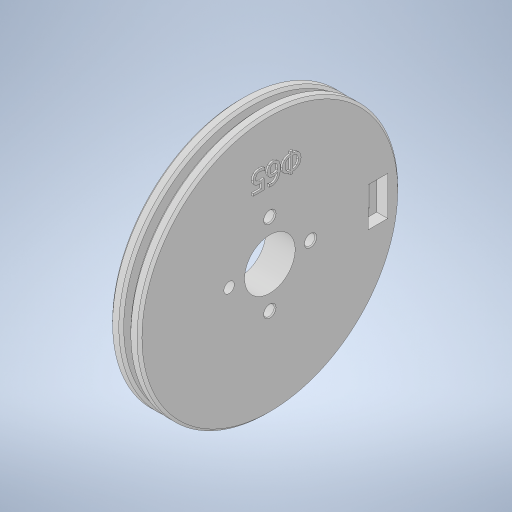
# Autodesk Inventor part: pully_elbow
Saved by Autodesk Inventor 2024 (Build 280153000, 153)
## iProperties
Created: 2025-06-10
Part Number: pully_elbow
Material: 一般
Document SubType Name: Modeling
Designer: HosodaLab2
Density: 1 g/cm^3
Appearance: 既定
Author: HosodaLab2
Autodesk Inventor part; units mm, degrees
ref_plane "YZ Plane" through (0, 0, 0) normal (1, 0, 0) x (0, 1, 0)
ref_plane "XZ Plane" through (0, 0, 0) normal (0, 1, 0) x (-1, 0, 0)
ref_plane "XY Plane" through (0, 0, 0) normal (0, 0, 1) x (1, 0, 0)
sketch "スケッチ1" plane through (0, 0, 0) normal (0, 1, 0) x (-1, 0, 0)
  circle A0 centre (0, 0) radius 32.5
  dimension "d0" = 65
  constraints: 1 centre point, 1 coincident
  measures "d0" diameter of A0
extrude "押し出し1" add sketch "スケッチ1" along normal blind 2.2
sketch "スケッチ2" plane through (0, 2.2, 0) normal (0, 1, 0) x (1, 0, 0)
  circle A0 centre (0, 0) radius 40
  line L0 (-3.103, -20.7113) -> (4.1548, -20.7113) construction
  line L1 (4.1548, -20.7113) -> (4.1548, -23.6986) construction
  line L2 (4.1548, -23.6986) -> (-3.103, -23.6986) construction
  line L3 (-3.103, -23.6986) -> (-3.103, -20.7113) construction
  dimension "d3" = 80
  constraints: 1 centre point, 1 coincident, 2 other
  measures "d3" diameter of A0
extrude "押し出し2" add sketch "スケッチ2" along normal blind 3.4
chamfer "面取り1" distance 0.75 angle 45 1 edges at (-40, 2.2, 0)
chamfer "面取り2" distance 0.75 angle 45 1 edges at (-40, 5.6, 0)
sketch "スケッチ3" plane through (0, 0, 0) normal (0, -1, 0) x (1, 0, 0)
  circle A0 centre (0, 0) radius 40
  dimension "d12" = 80
  constraints: 1 centre point, 1 coincident
  measures "d12" diameter of A0
extrude "押し出し3" add sketch "スケッチ3" along normal blind 3.4
chamfer "面取り3" distance 0.75 angle 45 1 edges at (-40, 0, 0)
chamfer "面取り4" distance 0.75 angle 45 1 edges at (-40, -3.4, 0)
sketch "スケッチ5" plane through (0, -3.4, 0) normal (0, -1, 0) x (1, 0, 0)
  circle A0 centre (0, 0) radius 12.5
  point P0 (0, -12.5)
  point P1 (0, 12.5)
  point P2 (-12.5, 0)
  point P3 (12.5, 0)
  dimension "d30" = 25
  constraints: 4 point on circle, 1 centre point, 1 coincident
  measures "d30" diameter of A0
hole "穴1" at (0, -3.4, -12.5) at (0, -3.4, 12.5) at (-12.5, -3.4, 0) at (12.5, -3.4, 0) direction (0, 1, 0) diameter 3.2 end through all
fillet "フィレット1" radius 0.3 6 edges at (0, -3.4, -10.9) (-12.5, -3.4, 1.6) (0, -3.4, 14.1) (0, 5.6, -10.9) (-12.5, 5.6, 1.6) (0, 5.6, 14.1)
sketch "スケッチ6" plane through (0, 5.6, 0) normal (0, 1, 0) x (1, 0, 0)
  circle A0 centre (0, 0) radius 3.15
  line L0 (0, 3.15) -> (39.8758, 3.15)
  circle A1 centre (0, 0) radius 40 projected
  line L1 (0, -3.15) -> (39.8758, -3.15)
  dimension "d39" = 6.3
  constraints: 4 end point, 4 point on circle, 1 centre point, 1 coincident, 1 horizontal, 1 parallel, 1 tangent
  measures "d39" diameter of A0
extrude "押し出し5" [suppressed]
chamfer "面取り7" [suppressed]
chamfer "面取り8" [suppressed]
chamfer "面取り9" [suppressed]
sketch "スケッチ7" plane through (0, 5.6, 0) normal (0, 1, 0) x (1, 0, 0)
  line L0 (-9.3358, -20.9354) -> (21.308, -20.9354) construction
  line L1 (21.308, -20.9354) -> (21.308, -27.5341) construction
  line L2 (21.308, -27.5341) -> (-9.3358, -27.5341) construction
  line L3 (-9.3358, -27.5341) -> (-9.3358, -20.9354) construction
  spline S0 degree 2 poles (-5.7914, -21.6472) (-5.2131, -21.6571) (-4.2541, -22.0427) (-3.9377, -22.364) knots 0 0 0 1 2 2 2
  spline S1 degree 2 poles (-3.9377, -22.364) (-3.646, -22.6655) (-3.3247, -23.5108) (-3.3247, -24.0546) knots 0 0 0 1 2 2 2
  spline S2 degree 2 poles (-3.3247, -24.0546) (-3.3247, -24.6231) (-3.6708, -25.498) (-3.9772, -25.7946) knots 0 0 0 1 2 2 2
  spline S3 degree 2 poles (-3.9772, -25.7946) (-4.3084, -26.1209) (-5.2773, -26.4818) (-5.7914, -26.4916) knots 0 0 0 1 2 2 2
  line L4 (-5.7914, -26.4916) -> (-5.7914, -27.1985)
  line L5 (-5.7914, -27.1985) -> (-6.6021, -27.1985)
  line L6 (-6.6021, -27.1985) -> (-6.6021, -26.4916)
  spline S4 degree 2 poles (-6.6021, -26.4916) (-7.1162, -26.4768) (-8.0802, -26.1407) (-8.4213, -25.8045) knots 0 0 0 1 2 2 2
  spline S5 degree 2 poles (-8.4213, -25.8045) (-8.7277, -25.503) (-9.0688, -24.6181) (-9.0688, -24.0546) knots 0 0 0 1 2 2 2
  spline S6 degree 2 poles (-9.0688, -24.0546) (-9.0688, -23.5207) (-8.7426, -22.6754) (-8.446, -22.369) knots 0 0 0 1 2 2 2
  spline S7 degree 2 poles (-8.446, -22.369) (-8.1296, -22.0427) (-7.1805, -21.6621) (-6.6021, -21.6472) knots 0 0 0 1 2 2 2
  line L7 (-6.6021, -21.6472) -> (-6.6021, -20.9997)
  line L8 (-6.6021, -20.9997) -> (-5.7914, -20.9997)
  line L9 (-5.7914, -20.9997) -> (-5.7914, -21.6472)
  spline S8 degree 2 poles (-5.7914, -25.8787) (-5.4207, -25.8688) (-4.8473, -25.6463) (-4.6594, -25.4585) knots 0 0 0 1 2 2 2
  spline S9 degree 2 poles (-4.6594, -25.4585) (-4.4073, -25.2113) (-4.17, -24.5044) (-4.17, -24.02) knots 0 0 0 1 2 2 2
  spline S10 degree 2 poles (-4.17, -24.02) (-4.17, -23.6147) (-4.3974, -22.9473) (-4.6248, -22.715) knots 0 0 0 1 2 2 2
  spline S11 degree 2 poles (-4.6248, -22.715) (-4.8374, -22.4925) (-5.4009, -22.28) (-5.7914, -22.2701) knots 0 0 0 1 2 2 2
  line L10 (-5.7914, -22.2701) -> (-5.7914, -25.8787)
  spline S12 degree 2 poles (-6.6021, -22.2701) (-6.9926, -22.275) (-7.5562, -22.4975) (-7.7687, -22.715) knots 0 0 0 1 2 2 2
  spline S13 degree 2 poles (-7.7687, -22.715) (-7.9961, -22.9424) (-8.2235, -23.6245) (-8.2235, -24.02) knots 0 0 0 1 2 2 2
  spline S14 degree 2 poles (-8.2235, -24.02) (-8.2235, -24.5044) (-7.9862, -25.2163) (-7.7341, -25.4585) knots 0 0 0 1 2 2 2
  spline S15 degree 2 poles (-7.7341, -25.4585) (-7.5463, -25.6365) (-6.9729, -25.8737) (-6.6021, -25.8787) knots 0 0 0 1 2 2 2
  line L11 (-6.6021, -25.8787) -> (-6.6021, -22.2701)
  spline S16 degree 2 poles (1.2428, -25.1718) (1.2428, -25.6414) (0.9314, -26.4373) (0.6694, -26.7042) knots 0 0 0 1 2 2 2
  spline S17 degree 2 poles (0.6694, -26.7042) (0.3975, -26.986) (-0.2846, -27.2776) (-0.6949, -27.2776) knots 0 0 0 1 2 2 2
  spline S18 degree 2 poles (-0.6949, -27.2776) (-1.1052, -27.2776) (-1.7824, -27.0008) (-2.0395, -26.724) knots 0 0 0 1 2 2 2
  spline S19 degree 2 poles (-2.0395, -26.724) (-2.3559, -26.3928) (-2.7118, -25.2805) (-2.7118, -24.4698) knots 0 0 0 1 2 2 2
  spline S20 degree 2 poles (-2.7118, -24.4698) (-2.7118, -23.674) (-2.3855, -22.3937) (-2.0444, -21.9191) knots 0 0 0 1 2 2 2
  spline S21 degree 2 poles (-2.0444, -21.9191) (-1.7132, -21.4544) (-0.6653, -20.9354) (0.0219, -20.9354) knots 0 0 0 1 2 2 2
  spline S22 degree 2 poles (0.0219, -20.9354) (0.2245, -20.9354) (0.5804, -20.9749) (0.7139, -21.0194) knots 0 0 0 1 2 2 2
  line L12 (0.7139, -21.0194) -> (0.7139, -21.8054)
  line L13 (0.7139, -21.8054) -> (0.6793, -21.8054)
  spline S23 degree 2 poles (0.6793, -21.8054) (0.5656, -21.7461) (0.1504, -21.6423) (-0.0869, -21.6423) knots 0 0 0 1 2 2 2
  spline S24 degree 2 poles (-0.0869, -21.6423) (-0.8482, -21.6423) (-1.7824, -22.6705) (-1.8714, -23.6789) knots 0 0 0 1 2 2 2
  spline S25 degree 2 poles (-1.8714, -23.6789) (-1.5798, -23.4762) (-0.9668, -23.2538) (-0.601, -23.2538) knots 0 0 0 1 2 2 2
  spline S26 degree 2 poles (-0.601, -23.2538) (-0.2451, -23.2538) (0.2888, -23.3972) (0.5804, -23.6147) knots 0 0 0 1 2 2 2
  spline S27 degree 2 poles (0.5804, -23.6147) (0.9166, -23.8668) (1.2428, -24.6478) (1.2428, -25.1718) knots 0 0 0 1 2 2 2
  spline S28 degree 2 poles (0.4124, -25.2064) (0.4124, -24.8307) (0.2146, -24.3215) (-0.0029, -24.1436) knots 0 0 0 1 2 2 2
  spline S29 degree 2 poles (-0.0029, -24.1436) (-0.166, -24.0151) (-0.5713, -23.931) (-0.7839, -23.931) knots 0 0 0 1 2 2 2
  spline S30 degree 2 poles (-0.7839, -23.931) (-1.0706, -23.931) (-1.6094, -24.104) (-1.8714, -24.2672) knots 0 0 0 1 2 2 2
  spline S31 degree 2 poles (-1.8714, -24.2672) (-1.8764, -24.3561) (-1.8862, -24.5242) (-1.8862, -24.6527) knots 0 0 0 1 2 2 2
  spline S32 degree 2 poles (-1.8862, -24.6527) (-1.8862, -25.2855) (-1.6391, -26.0616) (-1.4512, -26.2643) knots 0 0 0 1 2 2 2
  spline S33 degree 2 poles (-1.4512, -26.2643) (-1.2782, -26.457) (-0.9025, -26.6103) (-0.69, -26.6103) knots 0 0 0 1 2 2 2
  spline S34 degree 2 poles (-0.69, -26.6103) (-0.1956, -26.6103) (0.4124, -25.9083) (0.4124, -25.2064) knots 0 0 0 1 2 2 2
  spline S35 degree 2 poles (5.6621, -25.2113) (5.6621, -25.6513) (5.3804, -26.4027) (5.1233, -26.6795) knots 0 0 0 1 2 2 2
  spline S36 degree 2 poles (5.1233, -26.6795) (4.8663, -26.9563) (4.1001, -27.2776) (3.6255, -27.2776) knots 0 0 0 1 2 2 2
  spline S37 degree 2 poles (3.6255, -27.2776) (3.1905, -27.2776) (2.3403, -27.0848) (2.0288, -26.9316) knots 0 0 0 1 2 2 2
  line L14 (2.0288, -26.9316) -> (2.0288, -26.0665)
  line L15 (2.0288, -26.0665) -> (2.0881, -26.0665)
  spline S38 degree 2 poles (2.0881, -26.0665) (2.1821, -26.1357) (2.533, -26.3137) (2.7456, -26.3928) knots 0 0 0 1 2 2 2
  spline S39 degree 2 poles (2.7456, -26.3928) (2.9878, -26.4768) (3.3882, -26.5707) (3.6403, -26.5707) knots 0 0 0 1 2 2 2
  spline S40 degree 2 poles (3.6403, -26.5707) (3.8875, -26.5707) (4.3522, -26.3928) (4.5202, -26.2) knots 0 0 0 1 2 2 2
  spline S41 degree 2 poles (4.5202, -26.2) (4.6735, -26.0171) (4.8317, -25.5326) (4.8317, -25.2064) knots 0 0 0 1 2 2 2
  spline S42 degree 2 poles (4.8317, -25.2064) (4.8317, -24.8801) (4.6537, -24.4649) (4.4856, -24.3265) knots 0 0 0 1 2 2 2
  spline S43 degree 2 poles (4.4856, -24.3265) (4.3126, -24.1732) (3.7985, -24.0447) (3.4871, -24.0447) knots 0 0 0 1 2 2 2
  spline S44 degree 2 poles (3.4871, -24.0447) (3.151, -24.0447) (2.4836, -24.1485) (2.2809, -24.193) knots 0 0 0 1 2 2 2
  line L16 (2.2809, -24.193) -> (2.2809, -21.0491)
  line L17 (2.2809, -21.0491) -> (5.6275, -21.0491)
  line L18 (5.6275, -21.0491) -> (5.6275, -21.7659)
  line L19 (5.6275, -21.7659) -> (3.0669, -21.7659)
  line L20 (3.0669, -21.7659) -> (3.0669, -23.3922)
  spline S45 degree 2 poles (3.0669, -23.3922) (3.2152, -23.3724) (3.5019, -23.3576) (3.6206, -23.3576) knots 0 0 0 1 2 2 2
  spline S46 degree 2 poles (3.6206, -23.3576) (4.0902, -23.3576) (4.7377, -23.5108) (5.0343, -23.7382) knots 0 0 0 1 2 2 2
  spline S47 degree 2 poles (5.0343, -23.7382) (5.3359, -23.9656) (5.6621, -24.6577) (5.6621, -25.2113) knots 0 0 0 1 2 2 2
  point P0 (0, 0)
  constraints: 2 other
extrude "押し出し6" add sketch "スケッチ7" along normal blind 0.5
sketch "スケッチ8" plane through (0, 5.6, 0) normal (0, 1, 0) x (1, 0, 0)
  line L0 (-30.2, 6) -> (-36.2, 6)
  line L1 (-36.2, 6) -> (-36.2, -6)
  line L2 (-36.2, -6) -> (-30.2, -6)
  line L3 (-30.2, -6) -> (-30.2, 6)
  arc A0 (-32.5, 0) -> (-32.5, 0) centre (0, 0) ccw projected
  point P0 (-33.2, -6)
  point P1 (-33.2, 6)
  dimension "d53" = 12
  dimension "d54" = 6
  dimension "d55" = 30.2
  constraints: 8 end point, 2 midpoint, 2 parallel, 1 horizontal, 1 perpendicular
  measures "d53" distance of point (-33.2, -6) point (-33.2, 6)
  measures "d54" distance between parallel lines of L1 L3
  measures "d55" distance from line of point (0, 0) L3
extrude "押し出し7" cut sketch "スケッチ8" against normal blind 7.5 contours L3 L2 A0 L0 | A0 L2 L1 L0 picked at (-30.9459, 0.6701)
sketch "スケッチ9" plane through (0, 5.6, 0) normal (0, 1, 0) x (1, 0, 0)
  point P0 (0, 0)
  point P1 (0, 0)
  constraints: 1 coincident
hole "穴2" at (0, 5.6, 0) direction (0, -1, 0) diameter 15.5 end through all
